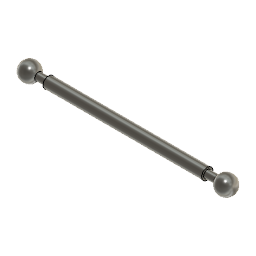
Benchwise base (Assembly) (Autodesk Fusion 360 archive; units mm, degrees)
design "screw base"
part number: 2026-04-16-17-30-08-607
Autodesk Fusion 360 part; units mm, degrees
cylinder "CylinderPrimitive1" add diameter 6 height 84 placed x (0, 0, -1) y (0, 1, 0) z (1, 0, 0) at (0, 0, 0)
sketch "Sketch2" plane through (0, 0, 0) normal (-1, 0, 0) x (0, -1, 0)
  circle A0 centre (0, 0) radius 3
  circle A1 centre (0, 0) radius 2
  dimension "d4" = 4
  constraint coincident A0.centre A1.centre
  measures "d4" diameter of A1
extrude "Extrude1" add sketch "Sketch2" along normal blind 10 contours A1
extrude "Extrude2" add 1 faces at (-10, -0.637, 0.1965) along direction (1, 0, 0) blind 10 from surface at 94
sphere "SpherePrimitive1" add diameter 10 placed x (0, -1, 0) y (0, 0, 1) z (-1, 0, 0) at (-10, 0, 0)
sphere "SpherePrimitive2" add diameter 10 placed x (0, 1, 0) y (0, 0, 1) z (1, 0, 0) at (94, 0, 0)

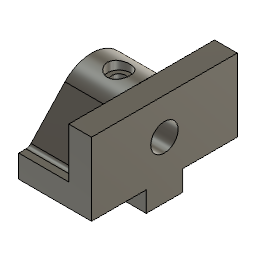
design "a"
part number: 2026-04-16-17-04-28-878
Autodesk Fusion 360 part; units mm, degrees
sketch "Sketch1" plane through (0, 0, 0) normal (1, 0, 0) x (0, 1, 0)
  line L0 (-11.5, 46) -> (-75.5, 46)
  line L1 (-75.5, 46) -> (-75.5, 14)
  line L2 (-11.5, 14) -> (-11.5, 46)
  line L3 (-11.5, 46) -> (-75.5, 14) construction
  line L4 (-75.5, 46) -> (-11.5, 14) construction
  line L5 (-35.5, 14) -> (-35.5, 5)
  line L6 (-35.5, 5) -> (-51.5, 5)
  line L7 (-51.5, 14) -> (-51.5, 5)
  line L8 (-43.5, 46) -> (-43.5, 14) construction
  circle A0 centre (-43.5, 30) radius 6
  line L9 (-11.5, 30) -> (-75.5, 30) construction
  line L10 (-11.5, 24) -> (-14.6971, 24)
  line L11 (-75.5, 24) -> (-72.3029, 24)
  line L12 (-16.8894, 24.9521) -> (-31.8079, 40.9222)
  line L13 (-70.1106, 24.9521) -> (-55.1921, 40.9222)
  arc A1 (-31.8079, 40.9222) -> (-55.1921, 40.9222) centre (-43.5, 30) ccw
  line L14 (-43.5, 5) -> (-43.5, 46) construction
  arc A2 (-16.8894, 24.9521) -> (-14.6971, 24) centre (-14.6971, 27) ccw
  arc A3 (-72.3029, 24) -> (-70.1106, 24.9521) centre (-72.3029, 27) ccw
  line L15 (-75.5, 14) -> (-51.5, 14)
  line L16 (-35.5, 14) -> (-11.5, 14)
  point P0 (-43.5, 30)
  point P1 (-16, 24)
  point P2 (-71, 24)
  dimension "d1" = 64
  dimension "d2" = 32
  dimension "d3" = 16
  dimension "d4" = 9
  dimension "d5" = 12
  dimension "d6" = 32
  dimension "d8" = 10
  dimension "d9" = 10
  dimension "d10" = 55
  dimension "d11" = 3
  constraint horizontal L0
  constraint perpendicular L0 L1
  constraint parallel L0 L15
  constraint parallel L1 L2
  constraint coincident L3 P0
  constraint coincident L4 P0
  constraint perpendicular L5 L16
  constraint perpendicular L2 L6
  constraint perpendicular L6 L7
  constraint midpoint L0 L8.start
  constraint symmetric L5 L7 L8
  constraint coincident L8 P0
  constraint concentric A0 A1
  constraint coincident P0 A0.centre
  constraint midpoint L2 L9.start
  constraint midpoint L1 L9.end
  constraint coincident L2 L10.start
  constraint perpendicular L2 L10
  constraint coincident L1 L11.start
  constraint perpendicular L1 L11
  constraint tangent L12 A1
  constraint tangent L13 A1
  constraint midpoint L6 L14.start
  constraint symmetric P1 P2 L14
  constraint coincident P1 L12
  constraint tangent L10 A2
  constraint tangent L12 A2
  constraint coincident P2 L11
  constraint coincident P2 L13
  constraint tangent L11 A3
  constraint tangent L13 A3
  constraint equal A2 A3
  constraint collinear L15 L16
  measures "d1" distance of L1.end L2.start
  measures "d2" distance of L0.end L1.end
  measures "d3" distance of L5.end L6.end
  measures "d4" distance of L6 L16
  measures "d5" diameter of A0
  measures "d6" diameter of A1
  measures "d8" distance of P2 L15
  measures "d9" distance of L2.start L10.start
  measures "d10" distance of P1 P2
  measures "d11" radius of A2
extrude "Extrude1" add sketch "Sketch1" against normal blind 24 contours L1 L2 L5 L6 L7 L10 L11 L12 L13 A1 A2 A3 L15 L16
extrude "Extrude2" cut 1 faces at (-24, -30.1612, 22.1163) along direction (1, 0, 0) blind 2
extrude "Extrude3" add sketch "Sketch1" against normal blind 10 contours L0 L2 L10 L12 A1 A2 | L0 L1 L11 L13 A1 A3
extrude "Extrude4" add sketch "Sketch1" against normal blind 32 contours L1 L2 L5 L6 L7 L10 L11 L12 L13 A1 A2 A3 L15 L16
sketch "Sketch3" plane through (0, 0, 5) normal (0, 0, -1) x (1, 0, 0)
  line L0 (-32, 35.5) -> (0, 35.5)
  line L1 (0, 35.5) -> (0, 51.5)
  line L2 (0, 51.5) -> (-32, 51.5)
  line L3 (-32, 51.5) -> (-32, 35.5)
  line L4 (0, 43.5) -> (-32, 43.5) construction
  line L5 (-16, 35.5) -> (-16, 51.5) construction
  line L6 (-8, 35.5) -> (-8, 51.5) construction
  line L7 (-24, 35.5) -> (-24, 51.5) construction
  circle A0 centre (-8, 43.5) radius 1 construction
  circle A1 centre (-24, 43.5) radius 1 construction
  dimension "d23" = 16
  dimension "d24" = 2
  dimension "d25" = 2
  constraint midpoint L1 L4.start
  constraint midpoint L3 L4.end
  constraint midpoint L0 L5.start
  constraint midpoint L2 L5.end
  constraint coincident L0 L6.start
  constraint coincident L2 L6.end
  constraint perpendicular L2 L6
  constraint coincident L0 L7.start
  constraint coincident L2 L7.end
  constraint perpendicular L2 L7
  constraint symmetric L5 L6 L7
  constraint midpoint L6 A0.centre
  constraint midpoint L7 A1.centre
  measures "d23" distance of L6 L7
  measures "d24" diameter of A0
  measures "d25" diameter of A1
hole "Hole1" at (-8, -43.5, 5) direction (0, 0, 1) diameter 6 depth 16 tip angle 100
hole "Hole2" at (-24, -43.5, 5) direction (0, 0, 1) diameter 6 depth 16 tip angle 100
sketch "Sketch4" plane through (0, 0, 46) normal (0, 0, 1) x (-1, 0, 0)
  line L0 (10, 43.5) -> (10, 75.5)
  line L1 (10, 75.5) -> (0, 75.5)
  line L2 (0, 75.5) -> (0, 11.5)
  line L3 (0, 11.5) -> (10, 11.5)
  line L4 (10, 11.5) -> (10, 43.5)
  line L5 (0, 43.5) -> (32, 43.5) construction
  line L6 (20, 50) -> (20, 38) construction
  line L7 (0, 11.5) -> (0, 75.5)
  circle A0 centre (20, 43.5) radius 1 construction
  dimension "d32" = 20
  dimension "d33" = 2
  constraint midpoint L2 L5.start
  constraint perpendicular L2 L5
  constraint perpendicular L5 L6
  constraint coincident L5 A0.centre
  constraint coincident L6 A0.centre
  measures "d32" distance of L6 L7
  measures "d33" diameter of A0
hole "Hole3" at (-20, -43.5, 46) direction (0, 0, -1) diameter 6 depth 12 tip angle 100 counterbore diameter 10 counterbore depth 4

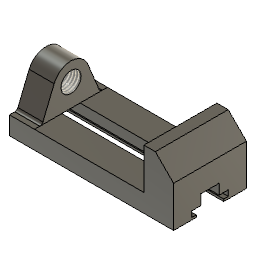
design "Benchwise base"
part number: 2026-04-16-16-12-37-495
Autodesk Fusion 360 part; units mm, degrees
sketch "Sketch1" plane through (0, 0, 0) normal (0, 0, 1) x (1, 0, 0)
  line L0 (-72, 32) -> (72, 32)
  line L1 (72, 32) -> (72, -32)
  line L2 (72, -32) -> (-72, -32)
  line L3 (-72, -32) -> (-72, 32)
  line L4 (-72, 32) -> (72, -32) construction
  line L5 (72, 32) -> (-72, -32) construction
  dimension "d1" = 144
  dimension "d2" = 64
  constraint horizontal L0
  constraint perpendicular L0 L1
  constraint parallel L0 L2
  constraint parallel L1 L3
  constraint coincident L4 origin
  constraint coincident L5 origin
  measures "d1" distance of L1.end L2.end
  measures "d2" distance of L0.end L1.end
extrude "Extrude1" add sketch "Sketch1" along normal blind 16
sketch "Sketch2" plane through (0, 0, 0) normal (0, 0, -1) x (1, 0, 0)
  line L0 (72, 32) -> (-72, 32)
  line L1 (-72, 32) -> (-72, -32)
  line L2 (-72, -32) -> (72, -32)
  line L3 (72, -32) -> (72, 32)
  line L4 (72, -16) -> (-72, -16)
  line L5 (-72, 16) -> (72, 16)
  line L6 (72, -8) -> (-72, -8)
  line L7 (-72, 8) -> (72, 8)
  line L8 (-72, 0) -> (72, 0) construction
  line L9 (72, -16) -> (72, -8)
  line L10 (72, 8) -> (72, 16)
  line L11 (-72, -16) -> (-72, -8)
  line L12 (-72, 8) -> (-72, 16)
  line L13 (-72, 12) -> (72, 12)
  line L14 (72, -12) -> (-72, -12)
  dimension "d5" = 16
  dimension "d6" = 32
  constraint coincident L3 L4.start
  constraint coincident L1 L4.end
  constraint perpendicular L1 L4
  constraint coincident L1 L5.start
  constraint coincident L3 L5.end
  constraint perpendicular L3 L5
  constraint coincident L3 L6.start
  constraint coincident L1 L6.end
  constraint perpendicular L1 L6
  constraint coincident L1 L7.start
  constraint coincident L3 L7.end
  constraint perpendicular L3 L7
  constraint midpoint L1 L8.start
  constraint midpoint L3 L8.end
  constraint symmetric L6 L7 L8
  constraint symmetric L4 L5 L8
  constraint midpoint L12 L13.start
  constraint midpoint L10 L13.end
  constraint midpoint L9 L14.start
  constraint midpoint L11 L14.end
  measures "d5" distance of L6 L7
  measures "d6" distance of L4 L5
extrude "Extrude2" cut sketch "Sketch2" against normal blind 7 contours L1 L3 L5 L10 L12 L13 | L1 L3 L7 L10 L12 L13 | L1 L3 L6 L9 L11 L14 | L1 L3 L4 L9 L11 L14
sketch "Sketch3" plane through (-72, 0, 0) normal (-1, 0, 0) x (0, -1, 0)
  line L0 (-8, 7) -> (-8, 0)
  line L1 (-8, 0) -> (8, 0)
  line L2 (8, 0) -> (8, 7)
  line L3 (8, 7) -> (16, 7)
  line L4 (16, 7) -> (16, 0)
  line L5 (16, 0) -> (32, 0)
  line L6 (32, 0) -> (32, 16)
  line L7 (32, 16) -> (-32, 16)
  line L8 (-32, 16) -> (-32, 0)
  line L9 (-32, 0) -> (-16, 0)
  line L10 (-16, 0) -> (-16, 7)
  line L11 (-16, 7) -> (-8, 7)
  circle A0 centre (0, 36) radius 8
  line L12 (32, 0) -> (14.8105, 42.0538) construction
  line L13 (-32, 0) -> (-14.8105, 42.0538) construction
  line L14 (0, 36) -> (16, 36) construction
  line L15 (0, 36) -> (-16, 36) construction
  arc A1 (14.8105, 42.0538) -> (-14.8105, 42.0538) centre (0, 36) ccw
  line L16 (32, 16) -> (32, 0) construction
  line L17 (0, 0) -> (0, 36) construction
  line L18 (14.8105, 42.0538) -> (24.6756, 17.9191)
  line L19 (-14.8105, 42.0538) -> (-24.6756, 17.9191)
  line L20 (-32, 16) -> (-27.4169, 16.0544)
  line L21 (32, 16) -> (27.4169, 16.0544)
  arc A2 (-27.4169, 16.0544) -> (-24.6756, 17.9191) centre (-27.4525, 19.0542) ccw
  arc A3 (24.6756, 17.9191) -> (27.4169, 16.0544) centre (27.4525, 19.0542) ccw
  dimension "d9" = 16
  dimension "d10" = 32
  dimension "d12" = 3
  dimension "d13" = 3
  dimension "d22" = 36
  constraint concentric A0 A1
  constraint coincident L5.end L6.start
  constraint tangent L12 A1
  constraint coincident L8.end L9.start
  constraint tangent L13 A1
  constraint coincident A0.centre L14.start
  constraint horizontal L14
  constraint parallel L14 L15
  constraint coincident L6.end L7.start
  constraint coincident L17.start origin
  constraint parallel L16 L17
  constraint coincident L7.end L8.start
  constraint tangent L19 A2
  constraint tangent L20 A2
  constraint tangent L18 A3
  constraint tangent L21 A3
  constraint coincident L12 L18.end
  constraint coincident L13 L19.end
  measures "d9" diameter of A0
  measures "d10" diameter of A1
  measures "d12" radius of A2
  measures "d13" radius of A3
  measures "d22" distance of L17.start A0.centre
extrude "Extrude3" add sketch "Sketch3" against normal blind 22 contours L7 A1 L18 L19 L20 L21 A2 A3
extrude "Extrude4" cut 1 faces at (-24, 2.6667, 0) along direction (0, 0, 1) blind 16
extrude "Extrude5" add sketch "Sketch2" against normal blind 2 contours L1 L3 L5 L10 L12 L13 | L1 L3 L4 L9 L11 L14
sketch "Sketch4" plane through (72, 0, 0) normal (1, 0, 0) x (0, 1, 0)
  line L0 (-8, 7) -> (-8, 16)
  line L1 (-8, 16) -> (-32, 16)
  line L2 (-32, 16) -> (-32, 0)
  line L3 (-32, 0) -> (-12, 0)
  line L4 (-12, 0) -> (-12, 2)
  line L5 (-12, 2) -> (-16, 2)
  line L6 (-16, 2) -> (-16, 7)
  line L7 (-16, 7) -> (-8, 7)
  line L8 (-32, 0) -> (32, 0)
  line L9 (32, 0) -> (32, 52)
  line L10 (32, 52) -> (-32, 52)
  line L11 (-32, 52) -> (-32, 0)
  line L12 (8, 16) -> (32, 16)
  line L13 (8, 16) -> (8, 7)
  line L14 (8, 7) -> (16, 7)
  line L15 (16, 7) -> (16, 2)
  line L16 (12, 2) -> (16, 2)
  line L17 (12, 0) -> (12, 2)
  line L18 (-32, 16) -> (-8, 16)
  line L19 (-8, 7) -> (-8, 16)
  line L20 (-16, 7) -> (-8, 7)
  line L21 (-16, 2) -> (-16, 7)
  line L22 (-16, 2) -> (-12, 2)
  line L23 (-12, 0) -> (-12, 2)
  line L24 (32, 0) -> (12, 0)
  line L25 (-12, 0) -> (-32, 0)
  line L26 (32, 16) -> (8, 16)
  line L27 (8, 7) -> (16, 7)
  line L28 (16, 2) -> (12, 2)
  line L29 (-8, 16) -> (8, 16)
  dimension "d20" = 64
  dimension "d21" = 52
  constraint horizontal L8
  constraint vertical L9
  constraint horizontal L10
  constraint vertical L11
  constraint coincident L2.end L3.start
  constraint coincident L12.end L26.start
  constraint coincident L12.start L13.start
  constraint coincident L13.end L14.start
  constraint coincident L14.end L15.start
  constraint coincident L15.end L16.end
  constraint coincident L16.start L17.end
  constraint coincident L0.end L1.start
  measures "d20" distance of L2.end L8.end
  measures "d21" distance of L2.end L10.end
extrude "Extrude6" add sketch "Sketch4" against normal blind 26 contours L0 L1 L2 L3 L4 L5 L6 L7 L8 L11 L18 L19 L20 L21 L22 L23 L25 | L1 L9 L10 L11 L12 L18 L26 L29 | L8 L9 L12 L13 L14 L15 L16 L17 L24 L26 L27 L28
chamfer "Chamfer1" distance 16 distance2 16 1 edges at (72, 0, 52) measured on face at (72, -2.6667, 40)
sketch "Sketch5" plane through (0, 0, 0) normal (0, 0, -1) x (1, 0, 0)
  line L0 (72, 32) -> (-72, 32)
  line L1 (-72, 32) -> (-72, 12)
  line L2 (-72, 12) -> (72, 12)
  line L3 (72, 12) -> (72, 32)
  line L4 (-72, 22) -> (72, 22) construction
  line L5 (72, -22) -> (-72, -22) construction
  line L6 (-35, 32) -> (-35, 12) construction
  line L7 (35, 32) -> (35, 12) construction
  line L8 (35.0796, -11.9043) -> (35.0796, -32) construction
  line L9 (-34.9204, -11.9904) -> (-34.9204, -32) construction
  line L10 (0, 32) -> (0, -32) construction
  line L11 (-71.7829, 0) -> (72, 0) construction
  circle A0 centre (35, 22) radius 2.5 construction
  circle A1 centre (-35, 22) radius 2.5 construction
  circle A2 centre (-34.9204, -21.9952) radius 2.5 construction
  circle A3 centre (35.0796, -21.9522) radius 2.5 construction
  dimension "d27" = 70
  dimension "d28" = 70
  dimension "d29" = 5
  dimension "d30" = 5
  dimension "d31" = 5
  dimension "d32" = 5
  constraint midpoint L1 L4.start
  constraint midpoint L3 L4.end
  constraint perpendicular L3 L5
  constraint coincident L0 L6.start
  constraint coincident L2 L6.end
  constraint perpendicular L2 L6
  constraint coincident L0 L7.start
  constraint coincident L2 L7.end
  constraint perpendicular L2 L7
  constraint perpendicular L5 L8
  constraint perpendicular L5 L9
  constraint midpoint L0 L10.start
  constraint perpendicular L5 L10
  constraint perpendicular L10 L11
  constraint symmetric L4 L5 L11
  constraint symmetric L6 L7 L10
  constraint midpoint L7 A0.centre
  constraint midpoint L6 A1.centre
  constraint midpoint L9 A2.centre
  constraint midpoint L8 A3.centre
  measures "d27" distance of L6 L7
  measures "d28" distance of L8 L9
  measures "d29" diameter of A0
  measures "d30" diameter of A1
  measures "d31" diameter of A2
  measures "d32" diameter of A3
hole "Hole1" at (-35, -22, 0) direction (0, 0, 1) diameter 6 depth 10 tip angle 118
pattern_linear "R-Pattern1" count 2 spacing 44 along (0, 1, 0) count 2 spacing 70 along (1, 0, 0) of "Hole1"
thread "Thread1" "ISO Metric profile 20.0 M20x2.5 M20x2.5 6H" major diameter 20.2925 minor diameter 17.519 pitch 2.5 angle 60 resizes the face on face at (-57.3333, -7.9901, 35.6012)
equation "d21 = 36 mm + 16 mm"

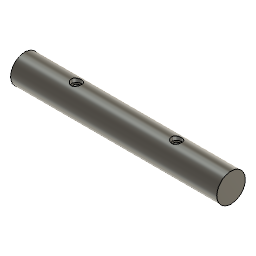
design "base plate"
part number: 2026-04-16-17-58-38-945
Autodesk Fusion 360 part; units mm, degrees
sketch "Sketch1" plane through (0, 0, 0) normal (1, 0, 0) x (0, 1, 0)
  circle A0 centre (0, 0) radius 10
  dimension "d1" = 20
  constraint coincident A0.centre origin
  measures "d1" diameter of A0
extrude "Extrude1" add sketch "Sketch1" along normal blind 144
sketch "Sketch2" plane through (0, 0, 0) normal (0, 0, 1) x (1, 0, 0)
  line L0 (0, 0) -> (144, 0) construction
  circle A0 centre (106, 0) radius 1
  circle A1 centre (36, 0) radius 1
  line L1 (106, 0, 0) -> (106, 0, 10.0443)
  line L2 (36, 0, 0) -> (36, 0, 10.2665)
  dimension "d4" = 2
  dimension "d5" = 2
  dimension "d6" = 144
  dimension "d7" = 38
  dimension "d8" = 70
  constraint coincident L0.start origin
  constraint horizontal L0
  constraint coincident L0 A0.centre
  constraint coincident L0 A1.centre
  measures "d4" diameter of A0
  measures "d5" diameter of A1
  measures "d6" distance of L0.start L0.end
  measures "d7" distance of L0.end A0.centre
  measures "d8" distance of A0.centre A1.centre
hole "Hole1" at (106, 0, 10.0443) direction (0, 0, -1) diameter 4 depth 7 tip angle 180 counterbore diameter 7 counterbore depth 3
pattern_linear "R-Pattern1" count 2 spacing 70 along (-1, 0, 0) of "Hole1"

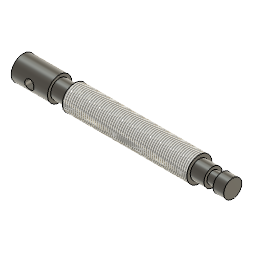
design "jow screw"
part number: 2026-04-16-17-38-59-076
Autodesk Fusion 360 part; units mm, degrees
sketch "Sketch1" plane through (0, 0, 0) normal (1, 0, 0) x (0, 1, 0)
  circle A0 centre (0, 0) radius 6
  circle A1 centre (0, 0) radius 4
  dimension "d1" = 12
  dimension "d2" = 8
  constraint coincident A0.centre A1.centre
  constraint concentric A0 A1
  measures "d1" diameter of A0
  measures "d2" diameter of A1
extrude "Extrude1" add sketch "Sketch1" along normal blind 7 contours A0 | A1 makes body 1
extrude "Extrude2" add sketch "Sketch1" against normal blind 6 contours A1 bodies 1
extrude "Extrude3" add sketch "Sketch1" against normal blind 9 from surface at -6 separate body makes body 2
extrude "Extrude4" add 1 faces at (-6, 1.4202, -0.5286) along direction (-1, 0, 0) blind 9 on bodies 1 bodies 1 2
sketch "Sketch2" plane through (-15, 0, 0) normal (-1, 0, 0) x (0, -1, 0)
  circle A0 centre (0, 0) radius 6
  circle A1 centre (0, 0) radius 8
  dimension "d12" = 16
  constraint coincident A0.centre A1.centre
  measures "d12" diameter of A1
extrude "Extrude5" add sketch "Sketch2" along normal blind 82 contours A0 | A1 bodies 1
sketch "Sketch3" plane through (-97, 0, 0) normal (-1, 0, 0) x (0, -1, 0)
  circle A0 centre (0, 0) radius 8
  circle A1 centre (0, 0) radius 6
  dimension "d15" = 12
  constraint coincident A0.centre A1.centre
  measures "d15" diameter of A1
extrude "Extrude6" add sketch "Sketch3" along normal blind 10 contours A1 bodies 1
sketch "Sketch4" plane through (-107, 0, 0) normal (-1, 0, 0) x (0, -1, 0)
  circle A0 centre (0, 0) radius 6
  circle A1 centre (0, 0) radius 8
  circle A2 centre (0, 0) radius 9
  dimension "d18" = 16
  dimension "d19" = 18
  constraint coincident A0.centre A1.centre
  measures "d18" diameter of A1
  measures "d19" diameter of A2
extrude "Extrude7" add sketch "Sketch4" along normal blind 24 contours A0 | A1 bodies 1
sketch "Sketch5" plane through (0, 0, 0) normal (0, 1, 0) x (1, 0, 0)
  line L0 (-107, 0) -> (-119, 0) construction
  circle A0 centre (-119, 0) radius 1 construction
  dimension "d22" = 2
  constraint horizontal L0
  constraint coincident L0.end A0.centre
  measures "d22" diameter of A0
hole "Hole1" at (-119, 0, 0) direction (0, -1, 0) diameter 6 depth 8 tip angle 180 bodies 1
extrude "Extrude8" cut 1 faces at (-117.6108, 0, -0.3851) along direction (0, 1, 0) blind 8 on bodies 1 bodies 1
thread "Thread1" "BSP Pipe Threads 3/8 G 3/8-19 G 3/8-19" major diameter 16.537 minor diameter 14.95 pitch 1.3368 angle 55 resizes the face on face at (-69.6667, -7.9901, -0.3988) on bodies 1
